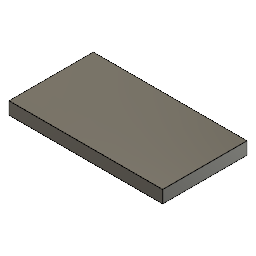
OpenBook Enclosure v6 (Autodesk Fusion 360 archive; units mm, degrees)
design "BATERIA"
Autodesk Fusion 360 part; units mm, degrees
box "BoxPrimitive1" add length 42 width 76.5 height 6.3 placed x (0, 0, 1) y (1, 0, 0) z (0, 1, 0) at (0, 0, 0)
